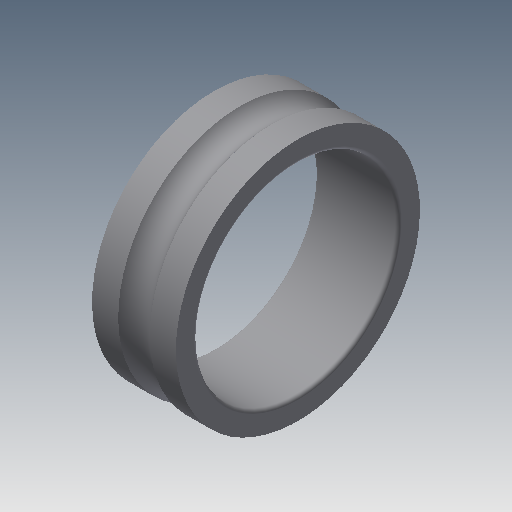
# Autodesk Inventor part: 676A Inner ring
Saved by Autodesk Inventor 2019.4 (Build 234330000, 330)
## iProperties
Category: PARTsolutions
Company: NTN
Created: 2019-06-11
Part Number: 676A Inner ring
Material: 一般
Catalog Web Link: www.cadenas.de
Description: Six types ir-Metric system sizes
Vendor: NTN
Document SubType Name: Modeling
Designer: psadmin
Manufacturer: NTN
Mass: 0.0299036 g
Surface Area: 1.31691 cm^2
Volume: 0.0299036 cm^3
Density: 1 g/cm^3
Appearance: PSOLRGB-192-192-192
PSOL_IDENT_0: {$CADENAS_DATA\23d-libs\ntn\ball_roller_bearings\miniature_extra_small_bb\metric_system_sizes\mss_ir
PSOL_IDENT_1: .prj},178 {VTYP=3D},{NB=676A Inner ring},{LINA=676A Inner ring},{NN=Six types ir},{DATE=29.01.2019 2
PSOL_IDENT_2: 3:03:31},{GEOMDATE=28.06.2007 12:57:00},{VERSION=},{LINEID=9710},{WBVAR=},{WBNUMERIC=}  {NB=676A Inn
PSOL_IDENT_3: er ring},{LINA=676A Inner ring},{KT=DUMMY},{IDNR=},{SD=6.0},{D=10},{B=2.5},{R=0.10},{ORDER=676A},{CR=
PSOL_IDENT_4: 465},{COR=196},{CRF=47},{CORF=20},{LSG=43 000},{LSO=51 000},{MASS=0.65},{D1=11.2},{D2=11.2},{C1=0.6}
PSOL_IDENT_5: ,{C2=0.6},{ORDER1=676A},{WSS=WA676AZ},{WDS=ZZ},{UTWF=FL676A},{FORSS=FLWA676AZ},{FORDS=ZZ},{DA1=6,6},
PSOL_IDENT_6: {DA2=6,7},{DA=9,2},{RAS=0,1},{MASS1=0.74},{B1=3.0},{VERS=1},{X=2},{N=12},{O=25.12},{RB=0.592}
NN: Six types ir
NT: Metric system sizes
NB: 676A Inner ring
NBSYN: $ORDER. Inner ring
LINA: 676A Inner ring
SD: 6
D: 10
B: 2.5
R: 0.1
CR: 465
COR: 196
CRF: 47
CORF: 20
LSG: 43 000
LSO: 51 000
MASS: 0.65
D1: 11.2
D2: 11.2
C1: 0.6
C2: 0.6
ORDER1: 676A
WSS: WA676AZ
WDS: ZZ
UTWF: FL676A
FORSS: FLWA676AZ
FORDS: ZZ
DA1: 6,6
DA2: 6,7
DA: 9,2
RAS: 0,1
MASS1: 0.74
B1: 3
VERS: 1
SUPPLIER: NTN
ARTICLENO: 676A Inner ring
BOMINFO: 676A Inner ring
CREATOR: CADENAS GmbH
Title: 676A Inner ring
Author: Cadenas PARTsolutions
Comments: Metric system sizes
Autodesk Inventor part; units mm, degrees
sketch "Sketch_1" plane through (0, 0, 0) normal (0, 0, 1) x (1, 0, 0)
  line L0 (2.5, 0) -> (0, 0)
  arc A0 (0, 3.1) -> (0.1, 3) centre (0.1, 3.1) ccw
  line L1 (0.1, 3) -> (2.4, 3)
  arc A1 (2.4, 3) -> (2.5, 3.1) centre (2.4, 3.1) ccw
  line L2 (2.5, 3.1) -> (2.5, 3.64)
  line L3 (2.5, 3.64) -> (1.72, 3.64)
  arc A2 (0.78, 3.64) -> (1.72, 3.64) centre (1.25, 4) ccw
  line L4 (0.78, 3.64) -> (0, 3.64)
  line L5 (0, 3.64) -> (0, 3.1)
  constraints: 12 end point, 6 point on circle, 3 centre point
revolve "Revolution1" add sketch "Sketch_1" angle 360 about axis through (2.5, 0, 0) along (1, 0, 0)
ref_plane "mss_ir_XY" through (0, 0, 0) normal (1, 0, 0) x (0, 0, -1)
ref_plane "mss_ir_YZ" through (0, 0, 0) normal (0, 0, -1) x (0, 1, 0)
ref_plane "mss_ir_ZX" through (0, 0, 0) normal (0, 1, 0) x (1, 0, 0)
body "Solid1"
